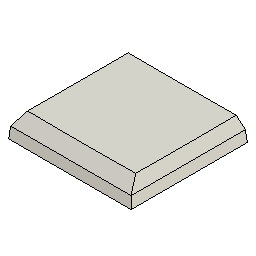
Choc v1 Cap v4 (Autodesk Fusion 360 design; units mm, degrees)
Autodesk Fusion 360 part; units mm, degrees
sketch "Base" plane through (0, 0, 0) normal (0, 0, 1) x (1, 0, 0)
  line L0 (8.8, -8.35) -> (-8.8, -8.35)
  line L1 (-8.8, -8.35) -> (-8.8, 8.35)
  line L2 (-8.8, 8.35) -> (8.8, 8.35)
  line L3 (8.8, 8.35) -> (8.8, -8.35)
  line L4 (8.8, -8.35) -> (-8.8, 8.35) construction
  line L5 (-8.8, -8.35) -> (8.8, 8.35) construction
  line L6 (13, 15) -> (14, 15)
  line L7 (8.6, 9.35) -> (-8.6, 9.35)
  line L8 (-9.8, 8.15) -> (-9.8, -8.15)
  line L9 (-8.6, -9.35) -> (8.6, -9.35)
  line L10 (9.8, -8.15) -> (9.8, 8.15)
  line L11 (9.8, 9.35) -> (-9.8, -9.35) construction
  line L12 (-9.8, 9.35) -> (9.8, -9.35) construction
  arc A0 (8.6, -9.35) -> (9.8, -8.15) centre (8.6, -8.15) ccw
  arc A1 (9.8, 8.15) -> (8.6, 9.35) centre (8.6, 8.15) ccw
  arc A2 (-8.6, 9.35) -> (-9.8, 8.15) centre (-8.6, 8.15) ccw
  arc A3 (-9.8, -8.15) -> (-8.6, -9.35) centre (-8.6, -8.15) ccw
  dimension "Depth" = 16.7
  dimension "Width" = 17.6
  dimension "OuterHoleGap" = 1
  dimension "d35" = 18.7
  dimension "d36" = 19.6
  dimension "d37" = 1.2
  constraint horizontal L0
  constraint perpendicular L0 L1
  constraint parallel L0 L2
  constraint parallel L1 L3
  constraint coincident L4 origin
  constraint coincident L5 origin
  constraint perpendicular L1 L6
  constraint horizontal L7
  constraint perpendicular L7 L8
  constraint parallel L7 L9
  constraint parallel L8 L10
  constraint coincident L11 origin
  constraint coincident L12 origin
  constraint coincident L12.end L9
  constraint coincident L12.end L10
  constraint tangent L9 A0
  constraint tangent L10 A0
  constraint coincident L11.start L10
  constraint coincident L11.start L7
  constraint tangent L10 A1
  constraint tangent L7 A1
  constraint equal A0 A1
  constraint coincident L12.start L7
  constraint coincident L12.start L8
  constraint tangent L7 A2
  constraint tangent L8 A2
  constraint equal A0 A2
  constraint coincident L11.end L8
  constraint coincident L11.end L9
  constraint tangent L8 A3
  constraint tangent L9 A3
  constraint equal A0 A3
  measures "Depth" distance of L0.start L2.end
  measures "Width" distance of L0.start L0.end
  measures "OuterHoleGap" distance of L6.start L6.end
  measures "d35" distance of L11.start L12.end
  measures "d36" distance of L11.start L12.start
  measures "d37" radius of A0
extrude "Extrude1" add sketch "Base" along normal blind 1.6 draft -5 contours L0 L1 L2 L3 makes body 1
extrude "Extrude2" add 1 faces at (-2.8867, -2.7367, 1.6) along direction (0, 0, 1) blind 1.8 separate body on bodies 1 makes body 2
draft "Draft1" angle -45 neutral plane through (0, 0, 1.6) pull (0, 0, -1) 1 faces at (2.8867, -8.21, 2.2) on bodies 2
draft "Draft2" angle -15 neutral plane through (0, 0, 1.6) pull (0, 0, -1) 1 faces at (-2.8867, 8.21, 2.2) on bodies 2
draft "Draft3" angle -30 neutral plane through (0, 0, 1.6) pull (0, 0, -1) 2 faces at (-8.66, -2.1367, 2.2) (8.66, -2.1367, 2.2) on bodies 2
sketch "Sketch8" plane through (0, 0, 0) normal (1, 0, 0) x (0, 1, 0)
  line L0 (-6.41, 3.4) -> (7.7277, 3.4)
  line L1 (0, 1.75) -> (0, 22.5)
  point P0 (0, 1003.4)
  dimension "TopR" = 1000
  constraint coincident P0 L1
  measures "TopR" distance of P0 L0
sphere "SpherePrimitive3" add diameter 2000 placed x (0, 1, 0) y (0, 0, 1) z (1, 0, 0) at (0, 0, 0) separate body makes body 3
move_body "Move1" bodies 3 to x (1, 0, 0) y (0, 1, 0) z (0, 0, 1) at (0, 0, 1003.1)
combine "Combine2" operation cut target body 2 tool bodies 3
combine "Combine3" operation add target body 1 tool bodies 2
shell "Shell1" thickness 0.7 removed faces 1 at (-2.9333, -2.7833, 0) on bodies 1
copy_body "CopyPasteBodies2" bodies 1 makes body 4
extrude "Extrude4" add 1 faces at (-2.6991, 8.1158, 0) along direction (0, 0, -1) blind 3 on bodies 4 bodies 4
fillet "Fillet2" radius 0.5 8 edges at (-8.8, -8.35, -1.5) (-8.73, -8.28, 0.8) (-8.8, 8.35, -1.5) (-8.73, 8.28, 0.8) (8.8, 8.35, -1.5) (8.73, 8.28, 0.8) (8.8, -8.35, -1.5) (8.73, -8.28, 0.8) on bodies 4
extrude "Extrude5" add sketch "Base" along normal blind 10 and the other way blind 3.3 separate body contours L0 L1 L2 L3 | L7 L8 L9 L10 A0 A1 A2 A3 makes body 5
copy_body "CopyPasteBodies3" bodies 5 makes body 6
copy_body "CopyPasteBodies1" bodies 1 makes body 7
sketch "Bump" plane through (0, 0, 0) normal (0, 0, 1) x (1, 0, 0)
  line L0 (2.5, -6.1) -> (-2.5, -6.1)
  line L1 (-2.5, -6.1) -> (-2.5, -5.9)
  line L2 (-2.5, -5.9) -> (2.5, -5.9)
  line L3 (2.5, -5.9) -> (2.5, -6.1)
  line L4 (2.5, -6.1) -> (-2.5, -5.9) construction
  line L5 (-2.5, -6.1) -> (2.5, -5.9) construction
  line L6 (0, 1.75) -> (0, 22.5)
  point P0 (0, -6)
  dimension "d21" = 0.2
  dimension "d22" = 5
  dimension "d23" = 6
  constraint horizontal L0
  constraint perpendicular L0 L1
  constraint parallel L0 L2
  constraint parallel L1 L3
  constraint coincident L4 P0
  constraint coincident L5 P0
  constraint coincident P0 L6
  measures "d21" distance of L0.start L2.end
  measures "d22" distance of L0.start L0.end
  measures "d23" distance of origin P0
extrude "Extrude3" add sketch "Bump" along normal blind 0.2 from the near side of the face at (4.3167, -0.2422, 3.1093) on bodies 7 bodies 7
move_body "Move2" bodies 1 5 7 4 6 to x (1, 0, 0) y (0, 1, 0) z (0, 0, 1) at (0, 0, 0)
hidden bodies 4 5 6 7
equation "FilletR = 0.2 mm"
equation "Travel = 3 mm"
equation "Thickness = 0.7 mm"
equation "StrokeTolerance = 0.3 mm"
equation "d33 = FilletR + StrokeTolerance"
equation "d35 = Depth + OuterHoleGap * 2"
equation "d36 = Width + OuterHoleGap * 2"
equation "d37 = FilletR + OuterHoleGap"
equation "d40 = Travel + StrokeTolerance"
equation "d45 = TopR * 2"
equation "d48 = TopR + 3.1 mm"
equation "LayoutAngle = 0.0 deg"
named bodies: "Placeholder", "Placeholder_Bump", "MEV", "Hole", "Territory"
